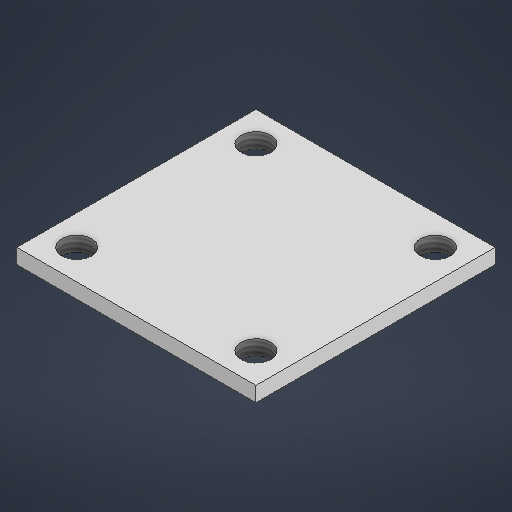
# Autodesk Inventor part: Top1
Saved by Autodesk Inventor 2026.1 (Build 301233000, 233)
## iProperties
Created: 2026-06-28
Part Number: Top1
Material: Generic
Document SubType Name: Modeling
Designer: Kasi Pusuluri
Density: 1 g/cm^3
Appearance: Default
Author: Kasi Pusuluri
Autodesk Inventor part; units mm, degrees
ref_plane "YZ Plane" through (0, 0, 0) normal (1, 0, 0) x (0, 1, 0)
ref_plane "XZ Plane" through (0, 0, 0) normal (0, 1, 0) x (-1, 0, 0)
ref_plane "XY Plane" through (0, 0, 0) normal (0, 0, 1) x (1, 0, 0)
sketch "Sketch1" plane through (0, 0, 0) normal (0, 1, 0) x (-1, 0, 0)
  line L0 (0, -25.4) -> (25.4, -25.4)
  line L1 (25.4, -25.4) -> (25.4, 25.4)
  line L2 (25.4, 25.4) -> (-25.4, 25.4)
  line L3 (25.4, 25.4) -> (-25.4, 25.4)
  line L4 (-25.4, 25.4) -> (-25.4, -25.4)
  line L5 (-25.4, -25.4) -> (25.4, -25.4)
  line L6 (25.4, -25.4) -> (25.4, 25.4)
  dimension "d6" = 50.8
  dimension "d7" = 50.8
  constraints: 14 end point, 3 horizontal, 2 parallel, 1 perpendicular, 1 vertical
  measures "d6" distance of L1.end L2.end
  measures "d7" distance of L3.end L4.end
extrude "Extrusion1" add sketch "Sketch1" along normal blind 3.175
sketch "Sketch3" plane through (0, 3.175, 0) normal (0, 1, 0) x (1, 0, 0)
  line L0 (0, 0) -> (-19.05, 0)
  line L1 (-19.05, 0) -> (-19.05, -19.05)
  line L2 (-19.05, -19.05) -> (0, -19.05)
  line L3 (0, -19.05) -> (0, 0)
  line L4 (-19.05, -19.05) -> (19.05, -19.05)
  line L5 (19.05, -19.05) -> (19.05, 19.05)
  line L6 (19.05, 19.05) -> (-19.05, 19.05)
  line L7 (-19.05, 19.05) -> (-19.05, -19.05)
  dimension "d8" = 19.05
  dimension "d9" = 19.05
  dimension "d10" = 38.1
  dimension "d11" = 38.1
  constraints: 16 end point, 4 coincident, 4 parallel, 2 horizontal, 2 perpendicular
  measures "d8" distance of L0.end L1.end
  measures "d9" distance of L1.end L2.end
  measures "d10" distance of L4.end L5.end
  measures "d11" distance of L5.end L6.end
hole "Hole1" at (-19.05, 3.175, 19.05) at (19.05, 3.175, 19.05) at (-19.05, 3.175, -19.05) at (19.05, 3.175, -19.05) at (19.05, 3.175, 19.05) direction (0, -1, 0) diameter 6.35 end through all
thread "Thread1" size "M6x1" class "6H" standard "ISO Metric profile" length 6.35
thread "Thread2" size "M6x1" class "6H" standard "ISO Metric profile" length 6.35
thread "Thread3" size "M6x1" class "6H" standard "ISO Metric profile" length 6.35
thread "Thread4" size "M6x1" class "6H" standard "ISO Metric profile" length 6.35
body "Solid1"
